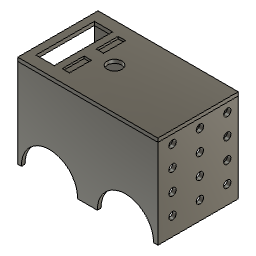
final_box v3 (Autodesk Fusion 360 design; units mm, degrees)
Autodesk Fusion 360 part; units mm, degrees
sketch "Sketch1" plane through (0, 0, 0) normal (0, 0, 1) x (1, 0, 0)
  line L0 (0, 0) -> (187, 0)
  line L1 (187, 0) -> (187, 100)
  line L2 (187, 100) -> (0, 100)
  line L3 (0, 100) -> (0, 0)
  line L4 (0, 0) -> (187, 0)
  line L5 (187, 0) -> (187, -5)
  line L6 (187, -5) -> (0, -5)
  line L7 (0, -5) -> (0, 0)
  line L8 (0, 100) -> (187, 100)
  line L9 (187, 100) -> (187, 105)
  line L10 (187, 105) -> (0, 105)
  line L11 (0, 105) -> (0, 100)
  line L12 (187, 105) -> (192, 105)
  line L13 (192, 105) -> (192, -5)
  line L14 (192, -5) -> (187, -5)
  line L15 (187, -5) -> (187, 105)
  dimension "d1" = 187
  dimension "d2" = 100
  dimension "d3" = 187
  dimension "d4" = 5
  dimension "d5" = 187
  dimension "d6" = 5
  dimension "d7" = 5
  constraint horizontal L0
  constraint vertical L1
  constraint horizontal L2
  constraint vertical L3
  constraint coincident L0.start L3.end
  constraint horizontal L4
  constraint vertical L5
  constraint horizontal L6
  constraint vertical L7
  constraint horizontal L8
  constraint vertical L9
  constraint horizontal L10
  constraint vertical L11
  constraint horizontal L12
  constraint vertical L13
  constraint horizontal L14
  constraint vertical L15
  measures "d1" distance of L0.start L0.end
  measures "d2" distance of L0.start L2.end
  measures "d3" distance of L0.start L0.end
  measures "d4" distance of L0.start L6.end
  measures "d5" distance of L2.end L1.end
  measures "d6" distance of L8 L10
  measures "d7" distance of L1 L13
extrude "Extrude1" add sketch "Sketch1" along normal blind 122 contours L0 L4 L5 L6 L7 L15 | L1 L5 L9 L12 L13 L14 L15 | L2 L8 L9 L10 L11 L15 makes body 1
sketch "Sketch2" plane through (187, 0, 0) normal (-1, 0, 0) x (0, -1, 0)
  line L0 (-100, 0) -> (0, 0)
  line L1 (0, 0) -> (0, 122)
  line L2 (0, 122) -> (-100, 122)
  line L3 (-100, 122) -> (-100, 0)
  line L4 (-105, 122) -> (5, 122)
  line L5 (5, 122) -> (5, 127)
  line L6 (5, 127) -> (-105, 127)
  line L7 (-105, 127) -> (-105, 122)
  dimension "d10" = 110
  dimension "d11" = 5
  constraint horizontal L4
  constraint vertical L5
  constraint horizontal L6
  constraint vertical L7
  measures "d10" distance of L4.start L4.end
  measures "d11" distance of L4.start L6.end
extrude "Extrude2" add sketch "Sketch2" along normal blind 192 separate body contours L2 L4 L5 L6 L7 makes body 2
move_body "Move1" bodies 2 to x (1, 0, 0) y (0, 1, 0) z (0, 0, 1) at (5, 0, 0)
sketch "Sketch3" plane through (192, 0, 0) normal (1, 0, 0) x (0, 1, 0)
  line L0 (-5, 0) -> (105, 0)
  line L1 (105, 0) -> (105, 122)
  line L2 (105, 122) -> (-5, 122)
  line L3 (-5, 122) -> (-5, 0)
  circle A0 centre (15, 110) radius 5
  circle A1 centre (52.5, 110) radius 5
  circle A2 centre (90, 110) radius 5
  circle A3 centre (15, 81.6667) radius 5
  circle A4 centre (52.5, 81.6667) radius 5
  circle A5 centre (90, 81.6667) radius 5
  circle A6 centre (15, 53.3333) radius 5
  circle A7 centre (52.5, 53.3333) radius 5
  circle A8 centre (90, 53.3333) radius 5
  circle A9 centre (15, 25) radius 5
  circle A10 centre (52.5, 25) radius 5
  circle A11 centre (90, 25) radius 5
  dimension "d14" = 10
  dimension "d17" = 75
  dimension "d18" = -85
  measures "d14" diameter of A0
extrude "Extrude3" cut sketch "Sketch3" against normal blind 10 contours A0 | A1 | A2 | A3 | A4 | A5 | A6 | A7 | A8 | A9 | A10 | A11 bodies 1
sketch "Sketch4" plane through (0, 0, 0) normal (-1, 0, 0) x (0, -1, 0)
  line L0 (-105, 0) -> (-100, 0)
  line L1 (-100, 0) -> (-100, 122)
  line L2 (-100, 122) -> (-105, 122)
  line L3 (-105, 122) -> (-105, 0)
  line L4 (-100, 64) -> (-85, 64)
  line L5 (-85, 64) -> (-85, 59)
  line L6 (-85, 59) -> (-100, 59)
  line L7 (-100, 59) -> (-100, 64)
  line L8 (0, 59) -> (-15, 59)
  line L9 (-15, 59) -> (-15, 64)
  line L10 (-15, 64) -> (0, 64)
  line L11 (0, 64) -> (0, 59)
  dimension "d21" = 15
  dimension "d22" = 5
  dimension "d23" = 58
  dimension "d24" = 15
  dimension "d25" = 5
  dimension "d26" = 58
  constraint horizontal L4
  constraint vertical L5
  constraint horizontal L6
  constraint vertical L7
  constraint coincident L1 L4.start
  constraint horizontal L8
  constraint vertical L9
  constraint horizontal L10
  constraint vertical L11
  measures "d21" distance of L4.start L4.end
  measures "d22" distance of L4.start L6.end
  measures "d23" distance of L2 L4
  measures "d24" distance of L8.start L8.end
  measures "d25" distance of L8.start L10.end
  measures "d26" distance of L2 L10
extrude "Extrude4" add sketch "Sketch4" against normal blind 185 contours L1 L4 L5 L6 L7 | L8 L9 L10 L11 bodies 1
sketch "Sketch5" plane through (0, 0, 127) normal (0, 0, 1) x (-1, 0, 0)
  line L0 (-192, 5) -> (-192, -105)
  line L1 (-192, -105) -> (0, -105)
  line L2 (0, -105) -> (0, 5)
  line L3 (0, 5) -> (-192, 5)
  line L4 (-10, -10) -> (-35, -10)
  line L5 (-35, -10) -> (-35, -90)
  line L6 (-35, -90) -> (-10, -90)
  line L7 (-10, -90) -> (-10, -10)
  dimension "d29" = 25
  dimension "d30" = 10
  constraint horizontal L4
  constraint vertical L5
  constraint horizontal L6
  constraint vertical L7
  measures "d29" distance of L5 L7
  measures "d30" distance of L2 L7
extrude "Extrude5" cut sketch "Sketch5" against normal blind 20 contours L4 L5 L6 L7 bodies 2
ref_plane "WorkPlane1" through (96, 50, 127) normal (0, 0, 1) x (0, 1, 0)
sketch "Sketch8" plane through (0, 0, 127) normal (0, 0, 1) x (1, 0, 0)
  circle A0 centre (75.7728, 51.7844) radius 10
  line L0 (44.0534, 88.4473) -> (54.0534, 88.4473)
  line L1 (54.0534, 88.4473) -> (54.0534, 58.4473)
  line L2 (54.0534, 58.4473) -> (44.0534, 58.4473)
  line L3 (44.0534, 58.4473) -> (44.0534, 88.4473)
  line L4 (54.0534, 88.4473) -> (54.0534, 58.4473)
  line L5 (44.0534, 41.7979) -> (54.0534, 41.7979)
  line L6 (54.0534, 41.7979) -> (54.0534, 11.7979)
  line L7 (54.0534, 11.7979) -> (44.0534, 11.7979)
  line L8 (44.0534, 11.7979) -> (44.0534, 41.7979)
  dimension "d39" = 20
  dimension "d40" = 10
  dimension "d41" = 30
  dimension "d42" = 10
  dimension "d43" = 30
  constraint horizontal L0
  constraint vertical L1
  constraint horizontal L2
  constraint vertical L3
  constraint vertical L4
  constraint horizontal L5
  constraint vertical L6
  constraint horizontal L7
  constraint vertical L8
  measures "d39" diameter of A0
  measures "d40" distance of L0.start L0.end
  measures "d41" distance of L0.start L2.end
  measures "d42" distance of L5.start L5.end
  measures "d43" distance of L5.start L7.end
extrude "Extrude6" cut sketch "Sketch8" against normal blind 60 contours A0 bodies 2
extrude "Extrude7" cut sketch "Sketch8" against normal blind 3 contours L5 L6 L7 L8 bodies 2
extrude "Extrude8" cut sketch "Sketch8" against normal blind 3 contours L0 L1 L2 L3 L4 bodies 2
ref_plane "WorkPlane2" through (96, -5, 61) normal (0, -1, 0) x (1, 0, 0)
sketch "Sketch9" plane through (0, -5, 0) normal (0, -1, 0) x (-1, 0, 0)
  circle A0 centre (-43.5076, -0.7615) radius 38.5
  circle A1 centre (-147.5475, -0.1904) radius 38.5
  dimension "d51" = 77
  dimension "d52" = 77
  measures "d51" diameter of A0
  measures "d52" diameter of A1
extrude "Extrude9" cut sketch "Sketch9" against normal blind 10000 bodies 1
